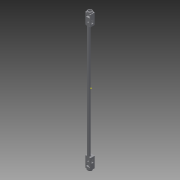
# Autodesk Inventor part: Axle280mm
Saved by Autodesk Inventor 2014 SP1 (Build 180222100, 222)
## iProperties
Created: 2017-01-06
Part Number: Axle280mm
Material: Generic
Document SubType Name: Modeling
Designer: danielsikar
Density: 1 g/cm^3
Appearance: Default
Author: danielsikar
Autodesk Inventor part; units mm, degrees
ref_plane "YZ Plane" through (0, 0, 0) normal (1, 0, 0) x (0, 1, 0)
ref_plane "XZ Plane" through (0, 0, 0) normal (0, 1, 0) x (-1, 0, 0)
ref_plane "XY Plane" through (0, 0, 0) normal (0, 0, 1) x (1, 0, 0)
sketch "Sketch1" plane through (0, 0, 0) normal (0, 0, 1) x (1, 0, 0)
  line L0 (0, 0) -> (4, 0)
  line L1 (4, 0) -> (4, 4)
  line L2 (4, 4) -> (0, 4)
  line L3 (0, 4) -> (0, 0)
  dimension "d0" = 4
  dimension "d1" = 4
  constraints: 8 end point, 2 parallel, 1 horizontal, 1 perpendicular
  measures "d0" distance of L2.end L1.end
  measures "d1" distance of L1.end L0.end
extrude "Extrusion1" add sketch "Sketch1" along normal blind 128.5
sketch "Sketch3" plane through (0, 0, 128.5) normal (0, 0, 1) x (1, 0, 0)
  line L0 (0, 0) -> (4, 0) projected
  line L1 (-3.5, 0) -> (7.5, 0)
  line L2 (7.5, 0) -> (7.5, 8)
  line L3 (7.5, 8) -> (-3.5, 8)
  line L4 (-3.5, 8) -> (-3.5, 0)
  point P0 (2, 0)
  dimension "d4" = 11
  dimension "d5" = 8
  constraints: 8 end point, 2 midpoint, 2 parallel, 1 horizontal, 1 perpendicular
  measures "d4" distance of L3.end L2.end
  measures "d5" distance of L2.end L1.end
extrude "Extrusion2" add sketch "Sketch3" along normal blind 11.5
sketch "Sketch4" plane through (0, 0, 0) normal (0, -1, 0) x (1, 0, 0)
  line L0 (7.5, 128.5) -> (7.5, 140) projected
  line L1 (-3.5, 140) -> (7.5, 140) projected
  line L2 (-1.75, 136) -> (5.75, 136)
  line L3 (5.75, 136) -> (5.75, 132.5)
  line L4 (5.75, 132.5) -> (-1.75, 132.5)
  line L5 (-1.75, 132.5) -> (-1.75, 136)
  point P0 (2, 136)
  point P1 (2, 140)
  point P2 (5.75, 134.25)
  point P3 (7.5, 134.25)
  dimension "d8" = 7.5
  dimension "d9" = 3.5
  constraints: 8 end point, 4 midpoint, 2 parallel, 1 horizontal, 1 horizontal alignment, 1 perpendicular, 1 vertical alignment
  measures "d8" distance of L3.end L4.end
  measures "d9" distance of L2.end L3.end
extrude "Extrusion3" cut sketch "Sketch4" against normal blind 8
sketch "Sketch5" plane through (0, 0, 140) normal (0, 0, 1) x (1, 0, 0)
  circle A0 centre (2, 4) radius 2.1
  point P0 (0, 0)
  dimension "d12" = 4.2
  constraints: 1 centre point
  measures "d12" diameter of A0
extrude "Extrusion4" cut sketch "Sketch5" against normal up to surface (7.5 mm away)
sketch "Sketch6" plane through (-3.5, 8, 128.5) normal (0, 1, 0) x (1, 0, 0)
  line L0 (11, 0) -> (0, 0) projected
  line L1 (0, 0) -> (0, -11.5) projected
  line L2 (11, -11.5) -> (0, -11.5) projected
  line L3 (11, 0) -> (11, -11.5) projected
  point P0 (3.5, 128.5)
extrude "Extrusion5" add sketch "Sketch6" along normal blind 1
mirror "Mirror2" about plane through (0, 0, 0) normal (0, 0, 1) of "Extrusion1", "Extrusion5", "Extrusion2", "Extrusion3", "Extrusion4"
sketch "Sketch7" plane through (0, 0, 140) normal (0, 0, 1) x (1, 0, 0)
  line L0 (-3.5, 0) -> (7.5, 0) projected
  arc A0 (4.0616, 0) -> (-0.0616, 0) centre (2, 4) ccw
  line L1 (0, 0) -> (-0.0616, 0)
  line L2 (-0.0616, 0) -> (4.0616, 0)
  circle A1 centre (2, 4) radius 3.25
  dimension "d17" = 9
  dimension "d18" = 6.5
  constraints: 4 end point, 2 centre point, 2 point on circle, 1 point on line
  measures "d17" diameter of A0
  measures "d18" diameter of A1
extrude "Extrusion6" add sketch "Sketch7" along normal blind 2.5
sketch "Sketch8" plane through (-3.5, 8, 128.5) normal (0, -1, 0) x (1, 0, 0)
  line L0 (1.75, 7.5) -> (1.75, 4) projected
  line L1 (1.75, 4) -> (9.25, 4) projected
  line L2 (9.25, 4) -> (9.25, 7.5) projected
  line L3 (9.25, 7.5) -> (1.75, 7.5) projected
  point P0 (3.5, -128.5)
mirror "Mirror3" about plane through (0, 0, 0) normal (0, 0, 1) of "Extrusion6"
sketch "Sketch10" plane through (-3.5, 9, -128.5) normal (0, 1, 0) x (1, 0, 0)
  line L0 (0, 0) -> (11, 0)
  line L1 (11, 0) -> (11, -9)
  line L2 (11, -9) -> (0, -9)
  line L3 (0, -9) -> (0, 0)
  point P0 (3.5, -128.5)
  dimension "d21" = 9
  constraints: 8 end point, 2 parallel, 1 horizontal, 1 perpendicular
  measures "d21" distance of L0.end L1.end
extrude "Extrusion7" add sketch "Sketch10" against normal up to surface (9 mm away)
sketch "Sketch11" plane through (-3.5, 9, -140) normal (0, 1, 0) x (1, 0, 0)
  line L0 (11, -20.5) -> (0, -20.5) projected
  circle A0 centre (5.5, -15) radius 2.1
  point P0 (3.5, -140)
  dimension "d24" = 4.2
  dimension "d25" = 5.5
  constraints: 1 centre point
  measures "d24" diameter of A0
  measures "d25" distance from line of A0.centre L0
extrude "Extrusion8" cut sketch "Sketch11" against normal blind 11
sketch "Sketch12" plane through (-3.5, 0, -140) normal (-1, 0, 0) x (0, 0, 1)
  line L0 (20.5, 9) -> (20.5, 0) projected
  line L1 (18.75, 6.25) -> (11.25, 6.25)
  line L2 (11.25, 6.25) -> (11.25, 2.75)
  line L3 (11.25, 2.75) -> (18.75, 2.75)
  line L4 (18.75, 2.75) -> (18.75, 6.25)
  point P0 (140, 0)
  point P1 (18.75, 4.5)
  point P2 (20.5, 4.5)
  dimension "d28" = 7.5
  dimension "d29" = 3.5
  dimension "d30" = 1.75
  constraints: 8 end point, 2 midpoint, 2 parallel, 1 horizontal, 1 horizontal alignment, 1 perpendicular
  measures "d28" distance of L3.end L2.end
  measures "d29" distance of L2.end L1.end
  measures "d30" distance between parallel lines of L0 L4
extrude "Extrusion9" cut sketch "Sketch12" against normal blind 11
fillet "Fillet3" radius 0.5 1 edges at (2, 8.5, -140)
sketch "Sketch14" plane through (-3.5, 9, -119.5) normal (0, 0, 1) x (1, 0, 0)
  line L0 (7.5, -9) -> (7.5, -5) projected
  line L1 (7.5, -9) -> (11, -9) projected
  line L2 (11, 0) -> (11, -9) projected
  line L3 (11, 0) -> (0, 0) projected
  line L4 (0, 0) -> (0, -9) projected
  line L5 (0, -9) -> (3.5, -9) projected
  line L6 (3.5, -5) -> (3.5, -9) projected
  line L7 (7.5, -5) -> (3.5, -5) projected
extrude "Extrusion10" add sketch "Sketch14" along normal blind 2
fillet "Fillet4" radius 1.5 3 edges at (4, 2, -117.5) (2, 4, -117.5) (0, 2, -117.5)
mirror "Mirror5" about plane through (0, 0, 0) normal (0, 0, 1) of "Extrusion7", "Extrusion8", "Extrusion9", "Extrusion10"
fillet "Fillet5" radius 1.5 3 edges at (0, 2, 117.5) (2, 4, 117.5) (4, 2, 117.5)
fillet "Fillet6" radius 0.5 1 edges at (2, 8.5, 140)
body "Solid1"
